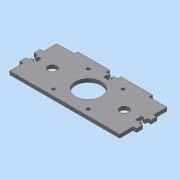
# Autodesk Inventor part: X-Motor-Housing_Front-Outer
Saved by Autodesk Inventor 2016 SP1 (Build 200210100, 210)
## iProperties
Created: 2015-12-01
Part Number: X-Motor-Housing_Front-Outer
Material: Generic
Document SubType Name: Modeling
Designer: Mohamed A.
Density: 1 g/cm^3
Appearance: Default
Mass: 9.53345 g
Surface Area: 82.3536 cm^2
Volume: 9.53345 cm^3
Author: Mohamed A.
Autodesk Inventor part; units mm, degrees
ref_plane "YZ Plane" through (0, 0, 0) normal (1, 0, 0) x (0, 1, 0)
ref_plane "XZ Plane" through (0, 0, 0) normal (0, 1, 0) x (-1, 0, 0)
ref_plane "XY Plane" through (0, 0, 0) normal (0, 0, 1) x (1, 0, 0)
sketch "Sketch12" plane through (0, 0, 0) normal (0, 0, 1) x (1, 0, 0)
  line L0 (-49, -21) -> (49, -21)
  line L1 (-49, 21) -> (-49, 9)
  line L2 (-49, -9) -> (-52, -9)
  line L3 (-52, -9) -> (-52, -3.75)
  line L4 (-52, 9) -> (-49, 9)
  line L5 (-49, -3.75) -> (-52, -3.75)
  line L6 (-49, 3.75) -> (-52, 3.75)
  line L7 (-44, -1.5) -> (-44, 1.5)
  line L8 (-49, 1.5) -> (-49, -1.5)
  line L9 (-49, -3.75) -> (-49, -9)
  line L10 (-49, 1.5) -> (-49, -1.5)
  line L11 (-49, 3.75) -> (-49, 1.5)
  line L12 (-47, -1.5) -> (-47, -2.65)
  line L13 (-44.6, -2.65) -> (-47, -2.65)
  line L14 (-44.6, -2.65) -> (-44.6, -1.5)
  line L15 (-44.6, 1.5) -> (-44.6, 2.65)
  line L16 (-47, 2.65) -> (-44.6, 2.65)
  line L17 (-47, 1.5) -> (-47, 2.65)
  line L18 (-49, -1.5) -> (-47, -1.5)
  line L19 (-44.6, -1.5) -> (-44, -1.5)
  line L20 (-44, 1.5) -> (-44.6, 1.5)
  line L21 (-47, 1.5) -> (-49, 1.5)
  line L22 (0, -30) -> (0, 33) construction
  line L23 (33.1667, 21) -> (33.1667, 24)
  line L24 (33.1667, 24) -> (5, 24)
  line L25 (-33.1667, 24) -> (-33.1667, 21)
  line L26 (-33.1667, 21) -> (-49, 21)
  line L27 (33.1667, 21) -> (49, 21)
  line L28 (-5, 21) -> (-5, 24)
  line L29 (5, 21) -> (5, 24)
  line L30 (-1.5, 21) -> (-1.5, 19)
  line L31 (-2.65, 19) -> (-1.5, 19)
  line L32 (-2.65, 19) -> (-2.65, 16.6)
  line L33 (-2.65, 16.6) -> (-1.5, 16.6)
  line L34 (-1.5, 16.6) -> (-1.5, 16)
  line L35 (-1.5, 16) -> (1.5, 16)
  line L36 (1.5, 16) -> (1.5, 16.6)
  line L37 (2.65, 16.6) -> (1.5, 16.6)
  line L38 (2.65, 16.6) -> (2.65, 19)
  line L39 (1.5, 19) -> (2.65, 19)
  line L40 (1.5, 19) -> (1.5, 21)
  line L41 (1.5, 21) -> (5, 21)
  line L42 (-5, 24) -> (-33.1667, 24)
  line L43 (5, 24) -> (-5, 24)
  line L44 (-1.5, 21) -> (-5, 21)
  circle A0 centre (0, 0) radius 11.5 projected
  circle A1 centre (32, 0) radius 3.9 projected
  circle A2 centre (-32, 0) radius 3.9 projected
  line L45 (2.65, 19) -> (2.65, 16.6) projected
  line L46 (2.65, 16.6) -> (-2.65, 16.6) projected
  line L47 (-2.65, 16.6) -> (-2.65, 19) projected
  line L48 (-2.65, 19) -> (2.65, 19) projected
  line L49 (44.6, 2.65) -> (47, 2.65) projected
  line L50 (47, 2.65) -> (47, -2.65) projected
  line L51 (47, -2.65) -> (44.6, -2.65) projected
  line L52 (44.6, -2.65) -> (44.6, 2.65) projected
  line L53 (-44.6, 2.65) -> (-44.6, -2.65) projected
  line L54 (-44.6, -2.65) -> (-47, -2.65) projected
  line L55 (-47, -2.65) -> (-47, 2.65) projected
  line L56 (-47, 2.65) -> (-44.6, 2.65) projected
  circle A3 centre (-15.5, -15.5) radius 1.4 projected
  circle A4 centre (-15.5, 15.5) radius 1.4 projected
  circle A5 centre (15.5, 15.5) radius 1.4 projected
  circle A6 centre (15.5, -15.5) radius 1.4 projected
  line L57 (-52, -21) -> (52, -21) projected
  line L58 (52, -21) -> (52, -10.5) projected
  line L59 (52, -10.5) -> (49, -10.5) projected
  line L60 (49, -10.5) -> (49, 10.5) projected
  line L61 (49, 10.5) -> (52, 10.5) projected
  line L62 (52, 10.5) -> (52, 24) projected
  line L63 (52, 24) -> (34.6667, 24) projected
  line L64 (34.6667, 24) -> (34.6667, 21) projected
  line L65 (34.6667, 21) -> (-34.6667, 21) projected
  line L66 (-34.6667, 21) -> (-34.6667, 24) projected
  line L67 (-34.6667, 24) -> (-52, 24) projected
  line L68 (-52, 24) -> (-52, 10.5) projected
  line L69 (-52, 10.5) -> (-49, 10.5) projected
  line L70 (-49, 10.5) -> (-49, -10.5) projected
  line L71 (-49, -10.5) -> (-52, -10.5) projected
  line L72 (-52, -10.5) -> (-52, -21) projected
  line L73 (-52, -3.75) -> (-52, 3.75)
  line L74 (-52, 3.75) -> (-52, 9)
  line L75 (-72.8, 0) -> (72.8, 0) construction
  line L76 (-49, -9) -> (-49, -21)
  line L77 (-49, 9) -> (-49, 3.75)
  line L78 (-49, -1.5) -> (-49, -3.75)
  line L79 (49, 21) -> (49, 9)
  line L80 (49, -9) -> (52, -9)
  line L81 (52, -9) -> (52, -3.75)
  line L82 (52, 9) -> (49, 9)
  line L83 (49, -3.75) -> (52, -3.75)
  line L84 (49, 3.75) -> (52, 3.75)
  line L85 (44, -1.5) -> (44, 1.5)
  line L86 (49, -3.75) -> (49, -9)
  line L87 (49, 1.5) -> (49, -1.5)
  line L88 (49, 3.75) -> (49, 1.5)
  line L89 (47, -1.5) -> (47, -2.65)
  line L90 (44.6, -2.65) -> (47, -2.65)
  line L91 (44.6, -2.65) -> (44.6, -1.5)
  line L92 (44.6, 1.5) -> (44.6, 2.65)
  line L93 (47, 2.65) -> (44.6, 2.65)
  line L94 (47, 1.5) -> (47, 2.65)
  line L95 (49, -1.5) -> (47, -1.5)
  line L96 (44.6, -1.5) -> (44, -1.5)
  line L97 (44, 1.5) -> (44.6, 1.5)
  line L98 (47, 1.5) -> (49, 1.5)
  line L99 (52, -3.75) -> (52, 3.75)
  line L100 (52, 3.75) -> (52, 9)
  line L101 (49, -9) -> (49, -21)
  line L102 (49, 9) -> (49, 3.75)
  line L103 (49, -1.5) -> (49, -3.75)
  point P0 (0, 0)
  dimension "d102" = 3
  dimension "d103" = 5
  dimension "d108" = 3
  dimension "d109" = 5
  dimension "d113" = 1.5
  dimension "d114" = 1.5
  dimension "d115" = 10
  dimension "d116" = 5.3
  dimension "d117" = 7.5
  constraints: 148 end point, 24 collinear, 16 perpendicular, 16 symmetric about line, 10 point on line, 5 parallel, 4 horizontal, 1 vertical, 7 other
  measures "d102" distance of L7.end L7.start
  measures "d103" distance between parallel lines of L8 L7
  measures "d108" distance between parallel lines of L36 L34
  measures "d109" distance between parallel lines of L41 L35
  measures "d113" distance between parallel lines of L2 L71
  measures "d114" distance between parallel lines of L25 L66
  measures "d115" distance between parallel lines of L29 L28
  measures "d116" distance between parallel lines of L32 L38
  measures "d117" distance between parallel lines of L6 L5
extrude "Extrusion9" add sketch "Sketch12" along normal blind 3 contours L76 L70 L9 L18 L12 L13 L14 L19 L7 L20 L15 L16 L17 L21 L11 L1 L26 L65 L44 L30 L31 L32 L33 L34 L35 L36 L37 L38 L39 L40 L41 L27 L79 L60 L98 L50 L49 L52 L97 L85 L96 L51 L95 L101 L0 | L2 L3 L5 L9 | L60 L83 L81 L80 | L74 L4 L70 L6 | L84 L60 L82 L100 | L96 L85 L97 L52 | L25 L42 L28 L65 | L65 L29 L24 L23
body "Solid3"
